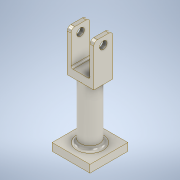
# Autodesk Inventor part: wheel connector
Saved by Autodesk Inventor 2022 (Build 260153000, 153)
## iProperties
Created: 2021-11-07
Part Number: wheel connector
Material: Titanium
Document SubType Name: Modeling
Designer: kibandi
Density: 4.51 g/cm^3
Appearance: Titanium
Mass: 2938.68 g
Surface Area: 798.687 cm^2
Volume: 651.591 cm^3
Author: kibandi
Autodesk Inventor part; units mm, degrees
ref_plane "YZ Plane" through (0, 0, 0) normal (1, 0, 0) x (0, 1, 0)
ref_plane "XZ Plane" through (0, 0, 0) normal (0, 1, 0) x (-1, 0, 0)
ref_plane "XY Plane" through (0, 0, 0) normal (0, 0, 1) x (1, 0, 0)
sketch "Sketch1" plane through (0, 0, 0) normal (0, 1, 0) x (-1, 0, 0)
  line L0 (0, 0) -> (100, 0)
  line L1 (100, 0) -> (100, -100)
  line L2 (100, -100) -> (0, -100)
  line L3 (0, -100) -> (0, 0)
  dimension "d0" = 100
  dimension "d1" = 100
  dimension "d2" = 100
  constraints: 8 end point, 2 perpendicular, 1 horizontal
  measures "d0" distance of L0.start L0.end
  measures "d1" distance of L0.end L1.end
  measures "d2" distance of L1.end L2.end
extrude "Extrusion1" add sketch "Sketch1" along normal blind 20
sketch "Sketch2" plane through (0, 20, 0) normal (0, 1, 0) x (1, 0, 0)
  line L0 (-100, 100) -> (-100, 0) projected
  line L1 (0, 100) -> (-100, 100) projected
  line L2 (-100, 0) -> (0, 0) projected
  circle A0 centre (-50, 50) radius 25
  dimension "d5" = 50
  constraints: 1 centre point
  measures "d5" diameter of A0
extrude "Extrusion2" add sketch "Sketch2" along normal blind 150
sketch "Sketch3" plane through (-50, 170, -50) normal (0, 1, 0) x (1, 0, 0)
  circle A0 centre (0, 0) radius 25 projected
  line L0 (0, 25) -> (35, 25)
  line L1 (35, 25) -> (35, -25)
  line L2 (0, 25) -> (-35, 25)
  line L3 (-35, 25) -> (-35, -25)
  line L4 (-35, -25) -> (35, -25)
  point P0 (50, -50)
  dimension "d12" = 35
  dimension "d13" = 35
  constraints: 10 end point, 4 horizontal, 2 perpendicular, 1 vertical alignment, 1 other
  measures "d12" distance of L0.start L0.end
  measures "d13" distance of L0.start L2.end
extrude "Extrusion3" add sketch "Sketch3" along normal blind 20
sketch "Sketch4" plane through (-50, 190, -50) normal (0, 1, 0) x (1, 0, 0)
  line L0 (0, 25) -> (-35, 25) projected
  line L1 (-35, 25) -> (-25, 25)
  line L2 (-25, 25) -> (-25, -25)
  line L3 (-35, -25) -> (0, -25) projected
  line L4 (-35, -25) -> (-35, 25)
  line L5 (35, 25) -> (0, 25) projected
  line L6 (35, 25) -> (25, 25)
  line L7 (25, 25) -> (25, -25)
  line L8 (0, -25) -> (35, -25) projected
  line L9 (35, -25) -> (35, 25)
  point P0 (50, -50)
  dimension "d14" = 10
  dimension "d15" = 10
  constraints: 12 end point, 4 point on line, 2 parallel, 2 perpendicular
  measures "d14" distance of L0.end L1.end
  measures "d15" distance of L5.start L6.end
extrude "Extrusion4" add sketch "Sketch4" along normal blind 90 contours L2 L3 L4 L0 | L5 L9 L8 L7
sketch "Sketch5" plane through (-75, 190, -25) normal (1, 0, 0) x (0, 0, -1)
  line L0 (50, 0) -> (50, 90) projected
  line L1 (0, -20) -> (0, 90) projected
  circle A0 centre (25, 70) radius 10
  line L2 (50, 90) -> (0, 90) projected
  point P0 (-25, -190)
  dimension "d20" = 20
  constraints: 1 centre point
  measures "d20" diameter of A0
sketch "Sketch6" plane through (-15, 170, -25) normal (1, 0, 0) x (0, 0, -1)
  line L0 (50, 20) -> (50, 110) projected
  line L1 (50, 110) -> (50, 70)
  circle A0 centre (25, 90) radius 10
  line L2 (0, 110) -> (50, 110) projected
  point P0 (-25, -170)
  dimension "d23" = 20
  constraints: 2 end point, 1 centre point, 1 point on line
  measures "d23" diameter of A0
extrude "Extrusion5" cut sketch "Sketch6" against normal blind 10
extrude "Extrusion6" cut sketch "Sketch5" against normal blind 10
fillet "Fillet1" radius 5 2 edges at (-25, 190, -50) (-75, 190, -50)
fillet "Fillet2" radius 10 4 edges at (-20, 280, -25) (-20, 280, -75) (-80, 280, -75) (-80, 280, -25)
fillet "Fillet3" radius 10 1 edges at (-75, 20, -50)
body "Solid1"
